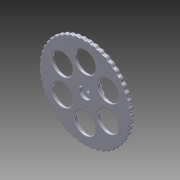
# Autodesk Inventor part: filter-wheel
Saved by Autodesk Inventor 2015 (Build 190159000, 159)
## iProperties
Created: 2014-09-28
Part Number: filter-wheel
Material: ABS Plastic
Document SubType Name: Modeling
Designer: Adam
Density: 1.06 g/cm^3
Appearance: Cool White
Author: Adam
Autodesk Inventor part; units mm, degrees
ref_plane "Work Plane1" through (0, 0, 0.25) normal (0, 0, 1) x (1, 0, 0)
sketch "Sketch2" plane through (0, 0, 0.25) normal (0, 0, 1) x (1, 0, 0)
  circle A0 centre (0, -28.75) radius 10 construction
  circle A1 centre (0, 0) radius 12.5 construction
  circle A2 centre (0, 0) radius 50
  spline S0 degree 3 poles (-30.5804, -41.1267) (-30.373, -40.8548) (-30.2921, -40.5013) (-30.2914, -39.6798) (-30.4245, -39.201) (-30.7705, -38.2638) (-30.9979, -37.7985) (-31.4911, -36.8888) (-31.7588, -36.4444) (-32.5953, -35.1256) (-33.1977, -34.2645) (-34.6466, -32.2338) (-35.5039, -31.0674) (-37.1953, -28.7098) (-38.028, -27.5218) (-38.8418, -26.3209) knots -1.739272 -1.739272 -1.739272 -1.739272 -1.636925 -1.636925 -1.492805 -1.492805 -1.337203 -1.337203 -1.181602 -1.181602 -0.870399 -0.870399 -0.435199 -0.435199 0 0 0 0 projected
  arc A3 (-30.5804, -41.1267) -> (30.5804, -41.1267) centre (0, 0) ccw projected
  spline S1 degree 3 poles (38.8418, -26.3209) (37.2781, -28.6284) (35.6252, -30.8742) (33.3647, -34.0268) (32.7265, -34.9308) (31.8379, -36.315) (31.5532, -36.7814) (31.0285, -37.7361) (30.7862, -38.2245) (30.4279, -39.1888) (30.2929, -39.6696) (30.291, -40.4962) (30.3715, -40.8528) (30.5804, -41.1267) knots -3.700846 -3.700846 -3.700846 -3.700846 -2.864619 -2.864619 -2.537069 -2.537069 -2.373294 -2.373294 -2.209519 -2.209519 -2.064656 -2.064656 -1.96155 -1.96155 -1.96155 -1.96155 projected
  arc A4 (38.8418, -26.3209) -> (-38.8418, -26.3209) centre (0, 0) ccw projected
  point P0 (0, 0)
  dimension "d1" = 100
  constraints: 1 centre point
  measures "d1" diameter of A2
extrude "Extrusion1" add sketch "Sketch2" along normal blind 4 contours A2 S1 A4 S0 | S0 A4 S1 A2
sketch "Sketch3" plane through (0, 0, 4.25) normal (0, 0, 1) x (1, 0, 0)
  circle A0 centre (0, 0) radius 50 construction
  circle A1 centre (0, -28.75) radius 10 construction
  circle A2 centre (0, -28.75) radius 11
  point P0 (0, 0)
  dimension "d4" = 1
  constraints: 1 centre point, 1 coincident
  measures "d4" radial gap between concentric circles of A1 A2
extrude "Extrusion2" cut sketch "Sketch3" against normal through all
pattern_circular "Circular Pattern1" count 6 over 360 about axis through (0, 0, 0.25) along (0, 0, 1) of "Extrusion2"
sketch "Sketch4" plane through (0, 0, 0.25) normal (0, 0, -1) x (-1, 0, 0)
  circle A0 centre (0, -28.75) radius 11 projected
  circle A1 centre (24.8982, -14.375) radius 11 projected
  circle A2 centre (24.8982, 14.375) radius 11 projected
  circle A3 centre (0, 28.75) radius 11 projected
  circle A4 centre (-24.8982, 14.375) radius 11 projected
  circle A5 centre (-24.8982, -14.375) radius 11 projected
  circle A6 centre (0, -28.75) radius 13
  point P0 (0, 0)
  dimension "d10" = 2
  constraints: 1 centre point, 1 coincident
  measures "d10" radial gap between concentric circles of A6 A0
extrude "Extrusion3" cut sketch "Sketch4" against normal blind 3 contours A6
pattern_circular "Circular Pattern2" count 6 over 360 about axis through (0, 0, 0.25) along (0, 0, 1) of "Extrusion3"
sketch "Sketch5" plane through (0, 0, 4.25) normal (0, 0, 1) x (1, 0, 0)
  circle A0 centre (0, 0) radius 50 construction
  circle A1 centre (0, -46.5) radius 3.5 construction
  line L0 (0, 0) -> (0, -50) construction
  line L1 (0, 0) -> (-50, 0) construction
  circle A2 centre (6.1978, -46.0851) radius 3.5 construction
  circle A3 centre (12.2851, -44.8478) radius 3.5 construction
  circle A4 centre (18.1531, -42.8102) radius 3.5 construction
  circle A5 centre (23.6972, -40.0087) radius 3.5 construction
  circle A6 centre (28.8184, -36.4932) radius 3.5 construction
  circle A7 centre (33.4253, -32.3264) radius 3.5 construction
  circle A8 centre (37.4358, -27.5829) radius 3.5 construction
  circle A9 centre (40.7782, -22.3471) radius 3.5 construction
  circle A10 centre (43.3929, -16.7125) radius 3.5 construction
  circle A11 centre (45.2333, -10.7796) radius 3.5 construction
  circle A12 centre (46.2665, -4.6544) radius 3.5 construction
  circle A13 centre (46.474, 1.5538) radius 3.5 construction
  circle A14 centre (45.8523, 7.7343) radius 3.5 construction
  circle A15 centre (44.4123, 13.7768) radius 3.5 construction
  circle A16 centre (42.1797, 19.5735) radius 3.5 construction
  circle A17 centre (39.1945, 25.0208) radius 3.5 construction
  circle A18 centre (35.5098, 30.0217) radius 3.5 construction
  circle A19 centre (31.1915, 34.4868) radius 3.5 construction
  circle A20 centre (26.3165, 38.3365) radius 3.5 construction
  circle A21 centre (20.972, 41.5021) radius 3.5 construction
  circle A22 centre (15.2532, 43.9271) radius 3.5 construction
  circle A23 centre (9.2621, 45.5682) radius 3.5 construction
  circle A24 centre (3.1059, 46.3962) radius 3.5 construction
  circle A25 centre (-3.1059, 46.3962) radius 3.5 construction
  circle A26 centre (-9.2621, 45.5682) radius 3.5 construction
  circle A27 centre (-15.2532, 43.9271) radius 3.5 construction
  circle A28 centre (-20.972, 41.5021) radius 3.5 construction
  circle A29 centre (-26.3165, 38.3365) radius 3.5 construction
  circle A30 centre (-31.1915, 34.4868) radius 3.5 construction
  circle A31 centre (-35.5098, 30.0217) radius 3.5 construction
  circle A32 centre (-39.1945, 25.0208) radius 3.5 construction
  circle A33 centre (-42.1797, 19.5735) radius 3.5 construction
  circle A34 centre (-44.4123, 13.7768) radius 3.5 construction
  circle A35 centre (-45.8523, 7.7343) radius 3.5 construction
  circle A36 centre (-46.474, 1.5538) radius 3.5 construction
  circle A37 centre (-46.2665, -4.6544) radius 3.5 construction
  circle A38 centre (-45.2333, -10.7796) radius 3.5 construction
  circle A39 centre (-43.3929, -16.7125) radius 3.5 construction
  circle A40 centre (-40.7782, -22.3471) radius 3.5 construction
  circle A41 centre (-37.4358, -27.5829) radius 3.5 construction
  circle A42 centre (-33.4253, -32.3264) radius 3.5 construction
  circle A43 centre (-28.8184, -36.4932) radius 3.5 construction
  circle A44 centre (-23.6972, -40.0087) radius 3.5 construction
  circle A45 centre (-18.1531, -42.8102) radius 3.5 construction
  circle A46 centre (-12.2851, -44.8478) radius 3.5 construction
  circle A47 centre (-6.1978, -46.0851) radius 3.5 construction
  arc A48 (-3.2067, -47.9025) -> (3.2067, -47.9025) centre (0, -46.5) ccw
  arc A49 (3.2067, -47.9025) -> (6.6643, -49.5539) centre (6.1978, -46.0851) ccw
  arc A50 (-6.6643, -49.5539) -> (-3.2067, -47.9025) centre (-6.1978, -46.0851) ccw
  arc A51 (-6.6643, -49.5539) -> (6.6643, -49.5539) centre (0, 0) ccw
  point P0 (0, 0)
  point P1 (0, -50)
  dimension "d17" = 7
  dimension "d22" = 360
  constraints: 51 centre point, 20 point on circle, 4 concentric, 4 end point, 2 tangent, 1 coincident, 1 horizontal, 1 perpendicular, 1 point on line, 95 other
  measures "d17" diameter of A1
extrude "Extrusion4" cut sketch "Sketch5" against normal through all
pattern_circular "Circular Pattern3" count 47 over 360 about axis through (0, 0, 0.25) along (0, 0, 1) of "Extrusion4"
fillet "Fillet1" radius 2 1 edges at (-3.2067, -47.9025, 2.25)
pattern_circular "Circular Pattern4" count 47 over 360 about axis through (0, 0, 0.25) along (0, 0, 1) of "Fillet1"
sketch "Sketch6" plane through (0, 0, 0.25) normal (0, 0, -1) x (-1, 0, 0)
  circle A0 centre (0, 0) radius 47
  circle A1 centre (0, 0) radius 50 construction
  arc A2 (49.2949, -0.5181) -> (49.1502, 3.8095) centre (46.474, 1.5538) ccw construction
  circle A3 centre (0, -28.75) radius 13 projected
  circle A4 centre (24.8982, -14.375) radius 13 projected
  circle A5 centre (24.8982, 14.375) radius 13 projected
  circle A6 centre (0, 28.75) radius 13 projected
  circle A7 centre (-24.8982, 14.375) radius 13 projected
  circle A8 centre (-24.8982, -14.375) radius 13 projected
  circle A9 centre (0, -28.75) radius 15
  circle A10 centre (24.8982, -14.375) radius 15
  circle A11 centre (24.8982, 14.375) radius 15
  circle A12 centre (0, 28.75) radius 15
  circle A13 centre (-24.8982, 14.375) radius 15
  circle A14 centre (-24.8982, -14.375) radius 15
  dimension "d33" = 3
  dimension "d34" = 2
  dimension "d35" = 2
  dimension "d36" = 2
  dimension "d37" = 2
  dimension "d38" = 2
  dimension "d39" = 2
  constraints: 8 centre point, 8 coincident, 1 tangent
  measures "d33" radial gap between concentric circles of A1 A0
  measures "d34" radial gap between concentric circles of A10 A4
  measures "d35" radial gap between concentric circles of A5 A11
  measures "d36" radial gap between concentric circles of A3 A9
  measures "d37" radial gap between concentric circles of A8 A14
  measures "d38" radial gap between concentric circles of A7 A13
  measures "d39" radial gap between concentric circles of A6 A12
extrude "Extrusion5" cut sketch "Sketch6" against normal up to surface (3 mm away) contours A0 | A9 A14 A13 A12 A11 A10
fillet "Fillet2" radius 2 12 edges at (-14.5915, -25.2732, 1.75) (-10.3067, -17.8518, 1.75) (14.5915, -25.2732, 1.75) (10.3067, -17.8518, 1.75) (29.183, 0, 1.75) (20.6134, 0, 1.75) (-29.183, 0, 1.75) (-20.6134, 0, 1.75) (-14.5915, 25.2732, 1.75) (-10.3067, 17.8518, 1.75) (14.5915, 25.2732, 1.75) (10.3067, 17.8518, 1.75)
fillet "Fillet3" radius 1 196 edges at (38.775, 31.2821, 4.25) (39.3963, 29.0274, 4.25) (42.5985, 25.8348, 4.25) (42.9138, 23.5174, 4.25) (45.6619, 19.9264, 4.25) (45.6655, 17.5877, 4.25) (47.9104, 13.6625, 4.25) (47.6022, 11.3442, 4.25) (49.304, 7.1548, 4.25) (48.6895, 4.8982, 4.25) (49.8177, 0.5194, 4.25) (48.908, -1.6352, 4.25) (49.4424, -6.1253, 4.25) (48.2536, -8.1394, 4.25) (48.1848, -12.6607, 4.25) (46.7382, -14.4983, 4.25) (46.0674, -18.9701, 4.25) (44.3888, -20.5986, 4.25) (43.1279, -24.9411, 4.25) (41.2472, -26.3312, 4.25) (39.4188, -30.4669, 4.25) (37.3695, -31.594, 4.25) (35.0062, -35.4491, 4.25) (32.825, -36.293, 4.25) (29.969, -39.7986, 4.25) (27.6948, -40.3443, 4.25) (24.3969, -43.438, 4.25) (22.0703, -43.6757, 4.25) (18.3895, -46.3022, 4.25) (16.052, -46.2277, 4.25) (12.0539, -48.3402, 4.25) (9.7472, -47.9547, 4.25) (5.5033, -49.5155, 4.25) (3.2685, -48.826, 4.25) (-1.1456, -49.8072, 4.25) (1.1456, -49.8072, 4.25) (-3.2685, -48.826, 4.25) (-6.6643, -49.5539, 4.25) (-9.7472, -47.9547, 4.25) (-14.2637, -47.7349, 4.25) (-16.052, -46.2277, 4.25) (-20.4989, -45.4078, 4.25) (-22.0703, -43.6757, 4.25) (-26.3682, -42.2704, 4.25) (-27.6948, -40.3443, 4.25) (-31.7671, -38.3787, 4.25) (-32.825, -36.293, 4.25) (-36.599, -33.8021, 4.25) (-37.3695, -31.594, 4.25) (-40.7778, -28.6223, 4.25) (-41.2472, -26.3312, 4.25) (-44.229, -22.9318, 4.25) (-44.3888, -20.5986, 4.25) (-46.8909, -16.8321, 4.25) (-46.7382, -14.4983, 4.25) (-48.716, -10.4319, 4.25) (-48.2536, -8.1394, 4.25) (-49.6717, -3.8457, 4.25) (-48.908, -1.6352, 4.25) (-49.7411, 2.8093, 4.25) (-48.6895, 4.8982, 4.25) (-48.9229, 9.414, 4.25) (-47.6022, 11.3442, 4.25) (-47.2316, 15.8508, 4.25) (-45.6655, 17.5877, 4.25) (-44.6974, 22.0047, 4.25) (-42.9138, 23.5174, 4.25) (-41.3657, 27.766, 4.25) (-39.3963, 29.0274, 4.25) (-37.2958, 33.0318, 4.25) (-35.1758, 34.0194, 4.25) (-32.5603, 37.7081, 4.25) (-30.3276, 38.4044, 4.25) (-27.2438, 41.7115, 4.25) (-24.9382, 42.104, 4.25) (-21.4411, 44.9705, 4.25) (-19.1038, 45.0523, 4.25) (-15.2558, 47.4271, 4.25) (-12.9285, 47.1966, 4.25) (-8.7983, 49.0373, 4.25) (-6.5224, 48.4987, 4.25) (-2.1837, 49.7725, 4.25) (0, 48.9353, 4.25) (4.4698, 49.6195, 4.25) (6.5224, 48.4987, 4.25) (11.0435, 48.581, 4.25) (12.9285, 47.1966, 4.25) (17.4202, 46.6755, 4.25) (19.1038, 45.0523, 4.25) (23.486, 43.9372, 4.25) (24.9382, 42.104, 4.25) (29.1327, 40.4148, 4.25) (30.3276, 38.4044, 4.25) (34.2595, 36.1712, 4.25) (35.1758, 34.0194, 4.25) (32.825, -36.293, 0.25) (29.969, -39.7986, 0.25) (27.6948, -40.3443, 0.25) (24.3969, -43.438, 0.25) (22.0703, -43.6757, 0.25) (18.3895, -46.3022, 0.25) (16.052, -46.2277, 0.25) (12.0539, -48.3402, 0.25) (9.7472, -47.9547, 0.25) (5.5033, -49.5155, 0.25) (3.2685, -48.826, 0.25) (-1.1456, -49.8072, 0.25) (1.1456, -49.8072, 0.25) (-3.2685, -48.826, 0.25) (-6.6643, -49.5539, 0.25) (-9.7472, -47.9547, 0.25) (-14.2637, -47.7349, 0.25) (-16.052, -46.2277, 0.25) (-20.4989, -45.4078, 0.25) (-22.0703, -43.6757, 0.25) (-26.3682, -42.2704, 0.25) (-27.6948, -40.3443, 0.25) (-31.7671, -38.3787, 0.25) (-32.825, -36.293, 0.25) (-36.599, -33.8021, 0.25) (-37.3695, -31.594, 0.25) (-40.7778, -28.6223, 0.25) (-41.2472, -26.3312, 0.25) (-44.229, -22.9318, 0.25) (-44.3888, -20.5986, 0.25) (-46.8909, -16.8321, 0.25) (-46.7382, -14.4983, 0.25) (-48.716, -10.4319, 0.25) (-48.2536, -8.1394, 0.25) (-49.6717, -3.8457, 0.25) (-48.908, -1.6352, 0.25) (-49.7411, 2.8093, 0.25) (-48.6895, 4.8982, 0.25) (-48.9229, 9.414, 0.25) (-47.6022, 11.3442, 0.25) (-47.2316, 15.8508, 0.25) (-45.6655, 17.5877, 0.25) (-44.6974, 22.0047, 0.25) (-42.9138, 23.5174, 0.25) (-41.3657, 27.766, 0.25) (-39.3963, 29.0274, 0.25) (-37.2958, 33.0318, 0.25) (-35.1758, 34.0194, 0.25) (-32.5603, 37.7081, 0.25) (-30.3276, 38.4044, 0.25) (-27.2438, 41.7115, 0.25) (-24.9382, 42.104, 0.25) (-21.4411, 44.9705, 0.25) (-19.1038, 45.0523, 0.25) (-15.2558, 47.4271, 0.25) (-12.9285, 47.1966, 0.25) (-8.7983, 49.0373, 0.25) (-6.5224, 48.4987, 0.25) (-2.1837, 49.7725, 0.25) (0, 48.9353, 0.25) (4.4698, 49.6195, 0.25) (6.5224, 48.4987, 0.25) (11.0435, 48.581, 0.25) (12.9285, 47.1966, 0.25) (17.4202, 46.6755, 0.25) (19.1038, 45.0523, 0.25) (23.486, 43.9372, 0.25) (24.9382, 42.104, 0.25) (29.1327, 40.4148, 0.25) (30.3276, 38.4044, 0.25) (34.2595, 36.1712, 0.25) (35.1758, 34.0194, 0.25) (38.775, 31.2821, 0.25) (39.3963, 29.0274, 0.25) (42.5985, 25.8348, 0.25) (42.9138, 23.5174, 0.25) (45.6619, 19.9264, 0.25) (45.6655, 17.5877, 0.25) (47.9104, 13.6625, 0.25) (47.6022, 11.3442, 0.25) (49.304, 7.1548, 0.25) (48.6895, 4.8982, 0.25) (49.8177, 0.5194, 0.25) (48.908, -1.6352, 0.25) (49.4424, -6.1253, 0.25) (48.2536, -8.1394, 0.25) (48.1848, -12.6607, 0.25) (46.7382, -14.4983, 0.25) (46.0674, -18.9701, 0.25) (44.3888, -20.5986, 0.25) (43.1279, -24.9411, 0.25) (41.2472, -26.3312, 0.25) (39.4188, -30.4669, 0.25) (37.3695, -31.594, 0.25) (35.0062, -35.4491, 0.25) (30.3982, 4.8487, 4.25) (11, 28.75, 4.25) (-19.3982, 23.9013, 4.25) (-30.3982, -4.8487, 4.25) (-11, -28.75, 4.25) (19.3982, -23.9013, 4.25)
sketch "Sketch10" plane through (0, -28.75, 3.25) normal (0, 0, -1) x (-1, 0, 0)
  circle A0 centre (24.8982, 43.125) radius 11 construction
  circle A1 centre (24.8982, 14.375) radius 11 construction
  circle A2 centre (-24.8982, 14.375) radius 11 construction
  circle A3 centre (0, 0) radius 11 construction
  circle A4 centre (-24.8982, 43.125) radius 11 construction
  circle A5 centre (0, 57.5) radius 11 construction
  line L0 (24.8982, 43.125) -> (0, 57.5) construction
  line L1 (-24.8982, 43.125) -> (0, 57.5) construction
  line L2 (-24.8982, 43.125) -> (-24.8982, 14.375) construction
  line L3 (-24.8982, 14.375) -> (0, 0) construction
  line L4 (0, 0) -> (24.8982, 14.375) construction
  line L5 (24.8982, 14.375) -> (24.8982, 43.125) construction
  line L6 (12.4491, 7.1875) -> (0, 28.75) construction
  line L7 (0, 28.75) -> (-12.4491, 7.1875) construction
  line L8 (0, 28.75) -> (-24.8982, 28.75) construction
  line L9 (0, 28.75) -> (-12.4491, 50.3125) construction
  line L10 (0, 28.75) -> (12.4491, 50.3125) construction
  line L11 (0, 28.75) -> (24.8982, 28.75) construction
  arc A6 (-7.7942, 42.25) -> (7.7942, 42.25) centre (0, 46.75) ccw
  arc A7 (-15.5885, 28.75) -> (-7.7942, 42.25) centre (-15.5885, 37.75) ccw
  arc A8 (-7.7942, 15.25) -> (-15.5885, 28.75) centre (-15.5885, 19.75) ccw
  arc A9 (7.7942, 15.25) -> (-7.7942, 15.25) centre (0, 10.75) ccw
  arc A10 (15.5885, 28.75) -> (7.7942, 15.25) centre (15.5885, 19.75) ccw
  arc A11 (7.7942, 42.25) -> (15.5885, 28.75) centre (15.5885, 37.75) ccw
  dimension "d53" = 9
  constraints: 24 end point, 15 tangent, 12 point on circle, 6 centre point, 6 midpoint, 3 parallel, 2 equal radius, 2 point on line, 1 vertical
  measures "d53" radius of A6
extrude "Extrusion8" add sketch "Sketch10" along normal blind 8.5
fillet "Fillet5" radius 1 6 edges at (-7.7942, 13.5, -1) (7.7942, 13.5, -1) (15.5885, 0, -1) (7.7942, -13.5, -1) (-7.7942, -13.5, -1) (-15.5885, 0, -1)
sketch "Sketch11" plane through (0, -28.75, -5.25) normal (0, 0, -1) x (-1, 0, 0)
  circle A0 centre (15.5885, 19.75) radius 11.5 construction
  circle A1 centre (0, 10.75) radius 11.5 construction
  circle A2 centre (-15.5885, 19.75) radius 11.5 construction
  circle A3 centre (-15.5885, 37.75) radius 11.5 construction
  circle A4 centre (0, 46.75) radius 11.5 construction
  circle A5 centre (15.5885, 37.75) radius 11.5 construction
  arc A6 (11.6654, 27.85) -> (6.6121, 19.0974) centre (15.5885, 19.75) ccw construction
  arc A7 (5.0533, 18.1974) -> (-5.0533, 18.1974) centre (0, 10.75) ccw construction
  arc A8 (-6.6121, 19.0974) -> (-11.6654, 27.85) centre (-15.5885, 19.75) ccw construction
  arc A9 (-11.6654, 29.65) -> (-6.6121, 38.4026) centre (-15.5885, 37.75) ccw construction
  arc A10 (-5.0533, 39.3026) -> (5.0533, 39.3026) centre (0, 46.75) ccw construction
  arc A11 (6.6121, 38.4026) -> (11.6654, 29.65) centre (15.5885, 37.75) ccw construction
  arc A12 (4.2148, 21.4498) -> (-4.2148, 21.4498) centre (0, 10.75) ccw
  arc A13 (-4.2148, 21.4498) -> (-8.4295, 28.75) centre (-15.5885, 19.75) ccw
  arc A14 (-8.4295, 28.75) -> (-4.2148, 36.0502) centre (-15.5885, 37.75) ccw
  arc A15 (-4.2148, 36.0502) -> (4.2148, 36.0502) centre (0, 46.75) ccw
  arc A16 (4.2148, 36.0502) -> (8.4295, 28.75) centre (15.5885, 37.75) ccw
  arc A17 (8.4295, 28.75) -> (4.2148, 21.4498) centre (15.5885, 19.75) ccw
  point P0 (0, 28.75)
  dimension "d61" = 2.5
  constraints: 24 point on circle, 12 centre point, 11 equal radius, 6 concentric
  measures "d61" radial gap between concentric circles of A1 A7
extrude "Extrusion9" cut sketch "Sketch11" against normal up to surface (8.5 mm away)
sketch "Sketch12" plane through (0, -28.75, -5.25) normal (0, 0, -1) x (-1, 0, 0)
  arc A0 (4.2148, 36.0502) -> (8.4295, 28.75) centre (15.5885, 37.75) ccw projected
  arc A1 (8.4295, 28.75) -> (4.2148, 21.4498) centre (15.5885, 19.75) ccw projected
  arc A2 (4.2148, 21.4498) -> (-4.2148, 21.4498) centre (0, 10.75) ccw projected
  arc A3 (-4.2148, 21.4498) -> (-8.4295, 28.75) centre (-15.5885, 19.75) ccw projected
  arc A4 (-8.4295, 28.75) -> (-4.2148, 36.0502) centre (-15.5885, 37.75) ccw projected
  arc A5 (-4.2148, 36.0502) -> (4.2148, 36.0502) centre (0, 46.75) ccw projected
  circle A6 centre (0, 28.75) radius 6.5
  constraints: 1 centre point, 1 coincident, 1 tangent
extrude "Extrusion10" add sketch "Sketch12" against normal up to surface (8.5 mm away) contours A0 A6 A5 | A0 A1 A6 | A6 A4 A5 | A6 A3 A4 | A1 A2 A6 | A6 A2 A3
sketch "Sketch13" plane through (0, 0, 3.25) normal (0, 0, -1) x (-1, 0, 0)
  circle A0 centre (0, 0) radius 3.4 projected
  circle A1 centre (0, 0) radius 6.5 projected
extrude "Extrusion11" add sketch "Sketch13" along normal up to surface (3 mm away)
sketch "Sketch14" plane through (0, -28.75, -5.25) normal (0, 0, -1) x (-1, 0, 0)
  arc A0 (-5.0533, 39.3026) -> (5.0533, 39.3026) centre (0, 46.75) ccw projected
  circle A1 centre (0, 28.75) radius 9
  circle A2 centre (0, 28.75) radius 6.5
  circle A3 centre (0, 28.75) radius 6.5 projected
  constraints: 2 centre point, 2 coincident, 1 concentric, 1 equal radius
ref_plane "Work Plane2" through (-56.5001, -15.1854, -6.5) normal (0, 0, 1) x (1, 0, 0)
extrude "Extrusion12" add sketch "Sketch14" along normal up to surface (1.25 mm away)
sketch "Sketch15" plane through (0, 0, 4.25) normal (0, 0, 1) x (1, 0, 0)
  circle A0 centre (0, 0) radius 6.5 projected
  circle A1 centre (0, 0) radius 6.5 construction
  circle A2 centre (0, 0) radius 3.4 construction
  circle A3 centre (0, 0) radius 3.4 construction
extrude "Extrusion13" cut sketch "Sketch15" against normal blind 3
sketch "Sketch16" plane through (0, 0, 0.25) normal (0, 0, -1) x (-1, 0, 0)
  circle A0 centre (0, 0) radius 3.1489 projected
  circle A1 centre (0, 0) radius 6.5 projected
extrude "Extrusion14" add sketch "Sketch16" along normal blind 2
sketch "Sketch17" plane through (0, 0, 1.25) normal (0, 0, 1) x (1, 0, 0)
  circle A0 centre (0, 0) radius 3.4 projected
  circle A1 centre (0, 0) radius 1.4 construction
  circle A2 centre (0, 0) radius 1.9
  point P0 (0, 0)
  dimension "d74" = 0.5
  constraints: 1 centre point, 1 coincident
  measures "d74" radial gap between concentric circles of A1 A2
ref_plane "Work Plane3" through (-3.4, -3.4, 0.25) normal (0, 0, 1) x (1, 0, 0)
extrude "Extrusion15" add sketch "Sketch17" against normal up to surface (1 mm away)
sketch "Sketch18" plane through (0, 0, -6.5) normal (0, 0, -1) x (-1, 0, 0)
  circle A0 centre (0, 0) radius 9 construction
  point P0 (0, 0)
  point P1 (-7.7942, 4.5)
  point P2 (7.7942, -4.5)
ref_plane "Work Plane4" through (7.7942, 4.5, -6.5) normal (-0.5, 0.866, 0) x (-0.866, -0.5, 0)
equation "\"d35\" = d34"
equation "\"d36\" = d34"
equation "\"d37\" = d34"
equation "\"d38\" = d34"
equation "\"d39\" = d34"
body "Solid1"
